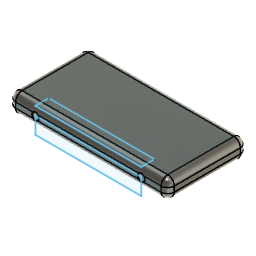
FloatIn v2 (Autodesk Fusion 360 design; units mm, degrees)
Autodesk Fusion 360 part; units mm, degrees
box "BoxPrimitive1" add length 120 width 240 height 28 placed x (0, 1, 0) y (-1, 0, 0) z (0, 0, 1) at (240, 0, 0)
fillet "Fillet1" radius 10 12 edges at (0, 60, 28) (0, 60, 0) (0, 0, 14) (120, 0, 28) (120, 0, 0) (240, 0, 14) (240, 60, 28) (240, 60, 0) (240, 120, 14) (120, 120, 0) (120, 120, 28) (0, 120, 14)
sketch "Sketch2" plane through (0, 0, 0) normal (0, -1, 0) x (1, 0, 0)
  line L0 (10, 18) -> (10, 10)
  line L1 (10, 10) -> (230, 10)
  line L2 (230, 10) -> (230, 18)
  line L3 (230, 18) -> (10, 18)
  line L4 (40, -10) -> (200, -10)
  line L5 (200, -10) -> (200, 15)
  line L6 (200, 15) -> (40, 15)
  line L7 (40, 15) -> (40, -10)
  dimension "d8" = 25
  constraint horizontal L4
  constraint vertical L5
  constraint horizontal L6
  constraint vertical L7
  measures "d8" distance of L4.start L6.end
sketch "Sketch3" plane through (0, 0, 0) normal (0, -1, 0) x (1, 0, 0)
  line L0 (40, 10) -> (42.6564, 10)
  line L1 (42.6564, 10) -> (42.6564, 14)
  line L2 (42.6564, 14) -> (40, 14)
  line L3 (40, 14) -> (40, 10)
  dimension "d9" = 4
  constraint horizontal L0
  constraint vertical L1
  constraint horizontal L2
  constraint vertical L3
  measures "d9" distance of L0.start L2.end
hole "Hole1" at (40, 0, 14) direction (0, 1, 0) diameter 10.2 depth 45 tip angle 118
sketch "Sketch4" plane through (0, 0, 0) normal (0, -1, 0) x (1, 0, 0)
  line L0 (200, 10) -> (206, 10)
  line L1 (206, 10) -> (206, 14)
  line L2 (206, 14) -> (200, 14)
  line L3 (200, 14) -> (200, 10)
  constraint horizontal L0
  constraint vertical L1
  constraint horizontal L2
  constraint vertical L3
hole "Hole2" at (200, 0, 14) direction (0, 1, 0) diameter 10.2 depth 45 tip angle 118
fillet "Fillet2" radius 0.5 8 edges at (45.1, 0, 14) (40, 0.0607, 8.9) (34.9, 0, 14) (40, 0.0607, 19.1) (194.9, 0, 14) (200, 0.0607, 19.1) (205.1, 0, 14) (200, 0.0607, 8.9)
sketch "Sketch5" plane through (0, 0, 28) normal (0, 0, 1) x (-1, 0, 0)
  line L0 (-230, -110) -> (-10, -110)
  line L1 (-10, -110) -> (-10, -10)
  line L2 (-10, -10) -> (-230, -10)
  line L3 (-230, -10) -> (-230, -110)
  line L4 (-40, 0) -> (-200, 0)
  line L5 (-200, 0) -> (-200, -20)
  line L6 (-200, -20) -> (-40, -20)
  line L7 (-40, -20) -> (-40, 0)
  constraint horizontal L4
  constraint vertical L5
  constraint horizontal L6
  constraint vertical L7
hole "Hole3" at (40.0901, 19.925, 28) direction (0, 0, -1) diameter 2 depth 14 tip angle 118
hole "Hole4" at (199.9487, 20.1464, 28) direction (0, 0, -1) diameter 2 depth 14 tip angle 118
